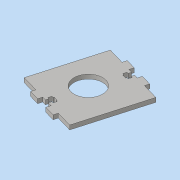
# Autodesk Inventor part: Part5
Saved by Autodesk Inventor 2016 SP1 (Build 200210100, 210)
## iProperties
Created: 2016-03-24
Part Number: Part5
Material: Generic
Document SubType Name: Modeling
Designer: Mohamed A.
Density: 1 g/cm^3
Appearance: Default
Author: Mohamed A.
Autodesk Inventor part; units mm, degrees
ref_plane "YZ Plane" through (0, 0, 0) normal (1, 0, 0) x (0, 1, 0)
ref_plane "XZ Plane" through (0, 0, 0) normal (0, 1, 0) x (-1, 0, 0)
ref_plane "XY Plane" through (0, 0, 0) normal (0, 0, 1) x (1, 0, 0)
sketch "Sketch1" plane through (0, 0, 0) normal (0, 0, 1) x (1, 0, 0)
  line L0 (-13.2512, -28.268) -> (-6.0407, -30.3316) projected
  line L1 (-6.0407, -30.3316) -> (-5.2152, -27.4474) projected
  circle A0 centre (-11.35, 0) radius 10.15 projected
  line L2 (-5.2152, -27.4474) -> (6.0812, -30.6803) projected
  line L3 (-28.3048, -23.9597) -> (-21.4231, -25.9292) projected
  line L4 (-21.4231, -25.9292) -> (-20.5977, -23.045) projected
  line L5 (-20.5977, -23.045) -> (-17.9538, -23.8017) projected
  line L6 (-17.9538, -23.8017) -> (-17.4035, -21.8789) projected
  line L7 (-17.4035, -21.8789) -> (-18.5091, -21.5624) projected
  line L8 (-18.5091, -21.5624) -> (-17.8488, -19.2551) projected
  line L9 (-17.8488, -19.2551) -> (-16.7432, -19.5715) projected
  line L10 (-16.7432, -19.5715) -> (-16.5781, -18.9947) projected
  line L11 (-16.5781, -18.9947) -> (-13.6939, -19.8201) projected
  line L12 (-13.6939, -19.8201) -> (-13.859, -20.3969) projected
  line L13 (-13.859, -20.3969) -> (-12.7534, -20.7134) projected
  line L14 (-12.7534, -20.7134) -> (-13.4137, -23.0207) projected
  line L15 (-13.4137, -23.0207) -> (-14.5193, -22.7043) projected
  line L16 (-14.5193, -22.7043) -> (-15.0696, -24.6271) projected
  line L17 (-15.0696, -24.6271) -> (-12.4258, -25.3838) projected
  line L18 (-12.4258, -25.3838) -> (-13.2512, -28.268) projected
  circle A1 centre (-11.35, 0) radius 13.25 projected
  line L19 (6.0812, -30.6803) -> (19.6734, 16.813) projected
  line L20 (19.6734, 16.813) -> (8.377, 20.0459) projected
  line L21 (8.377, 20.0459) -> (9.2024, 22.9301) projected
  line L22 (9.2024, 22.9301) -> (1.9919, 24.9937) projected
  line L23 (1.9919, 24.9937) -> (1.1664, 22.1095) projected
  line L24 (1.1664, 22.1095) -> (-1.4774, 22.8662) projected
  line L25 (-1.4774, 22.8662) -> (-2.0277, 20.9434) projected
  line L26 (-2.0277, 20.9434) -> (-0.9221, 20.627) projected
  line L27 (-0.9221, 20.627) -> (-1.5824, 18.3196) projected
  line L28 (-1.5824, 18.3196) -> (-2.6881, 18.636) projected
  line L29 (-2.6881, 18.636) -> (-2.8531, 18.0592) projected
  line L30 (-2.8531, 18.0592) -> (-5.7373, 18.8846) projected
  line L31 (-5.7373, 18.8846) -> (-5.5723, 19.4614) projected
  line L32 (-5.5723, 19.4614) -> (-6.6779, 19.7779) projected
  line L33 (-6.6779, 19.7779) -> (-6.0175, 22.0852) projected
  line L34 (-6.0175, 22.0852) -> (-4.9119, 21.7688) projected
  line L35 (-4.9119, 21.7688) -> (-4.3616, 23.6916) projected
  line L36 (-4.3616, 23.6916) -> (-7.0055, 24.4483) projected
  line L37 (-7.0055, 24.4483) -> (-6.18, 27.3325) projected
  line L38 (-6.18, 27.3325) -> (-13.0618, 29.302) projected
  line L39 (-13.0618, 29.302) -> (-13.8872, 26.4178) projected
  line L40 (-13.8872, 26.4178) -> (-25.5125, 29.7448) projected
  line L41 (-25.5125, 29.7448) -> (-39.1047, -17.7485) projected
  line L42 (-39.1047, -17.7485) -> (-27.4794, -21.0755) projected
  line L43 (-27.4794, -21.0755) -> (-28.3048, -23.9597) projected
  point P0 (0, 0)
extrude "Extrusion1" add sketch "Sketch1" along normal blind 3 contours L18 L17 L16 L15 L14 L13 L12 L11 L10 L9 L8 L7 L6 L5 L4 L3 L43 L42 L41 L40 L39 L38 L37 L36 L35 L34 L33 L32 L31 L30 L29 L28 L27 L26 L25 L24 L23 L22 L21 L20 L19 L2 L1 L0 | A1
body "Solid1"
